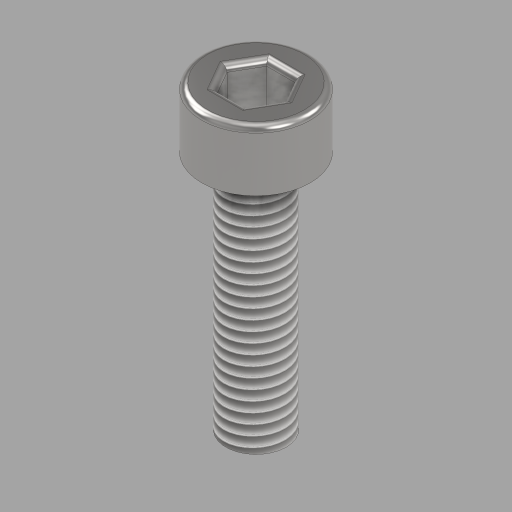
# Autodesk Inventor part: Screw_M4X12_SS_HEX
Saved by Autodesk Inventor 2024 (Build 280153020, 153B)
## iProperties
Created: 2023-06-02
Part Number: Screw_M4X12_SS_HEX
Material: Stainless Steel
Document SubType Name: Modeling
Designer: schanen
Density: 8 g/cm^3
Appearance: Semi-Polished
Author: schanen
Autodesk Inventor part; units mm, degrees
ref_plane "YZ Plane" through (0, 0, 0) normal (1, 0, 0) x (0, 1, 0)
ref_plane "XZ Plane" through (0, 0, 0) normal (0, 1, 0) x (-1, 0, 0)
ref_plane "XY Plane" through (0, 0, 0) normal (0, 0, 1) x (1, 0, 0)
sketch "Sketch1" plane through (0, 0, 0) normal (0, 0, 1) x (1, 0, 0)
  line L0 (0, 0) -> (0, 15)
  line L1 (0, 15) -> (-2.7, 15)
  line L2 (-2.7, 15) -> (-2.7, 12)
  line L3 (-2.7, 12) -> (-1.5, 12)
  line L4 (-1.5, 12) -> (-1.5, 0)
  line L5 (-1.5, 0) -> (0, 0)
  dimension "d0" = 12
  dimension "d1" = 3
  dimension "d2" = 1.5
  dimension "d3" = 2.7
  constraints: 12 end point, 5 perpendicular, 1 vertical
  measures "d0" distance of L3.end L4.end
  measures "d1" distance of L1.end L2.end
  measures "d2" distance of L4.end L0.start
  measures "d3" distance of L0.end L1.end
revolve "Revolution1" add sketch "Sketch1" angle 360 about axis through (0, 0, 0) along (0, 1, 0)
sketch "Sketch2" plane through (0, 15, 0) normal (0, 1, 0) x (1, 0, 0)
  line L0 (-0.7217, -1.25) -> (-1.4434, 0)
  line L1 (-1.4434, 0) -> (-0.7217, 1.25)
  line L2 (-0.7217, 1.25) -> (0.7217, 1.25)
  line L3 (0.7217, 1.25) -> (1.4434, 0)
  line L4 (1.4434, 0) -> (0.7217, -1.25)
  line L5 (0.7217, -1.25) -> (-0.7217, -1.25)
  point P0 (0, 0)
  point P1 (0, 0)
  dimension "d5" = 2.5
  constraints: 12 end point, 1 coincident, 1 horizontal alignment, 13 other
  measures "d5" distance between parallel lines of L2 L5
extrude "Extrusion1" cut sketch "Sketch2" against normal blind 2
fillet "Fillet1" radius 0.3 6 edges at (0, 15, -1.25) (1.0825, 15, -0.625) (1.0825, 15, 0.625) (0, 15, 1.25) (-1.0825, 15, 0.625) (-1.0825, 15, -0.625)
fillet "Fillet2" radius 0.3 1 edges at (2.7, 15, 0)
thread "Thread1" size "M3x0.5" class "6g" standard "ANSI Metric M Profile" length 11.5
body "Solid1"
